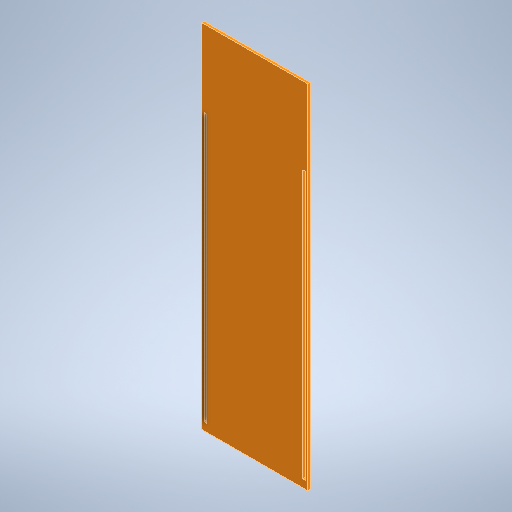
# Autodesk Inventor part: lifting cover 2
Saved by Autodesk Inventor 2025.4 (Build 294407000, 407)
## iProperties
Created: 2026-04-06
Part Number: lifting cover 2
Material: Generic
Document SubType Name: Modeling
Designer: abdo2
Density: 1 g/cm^3
Appearance: Orange
Author: abdo2
Autodesk Inventor part; units mm, degrees
ref_plane "YZ Plane" through (0, 0, 0) normal (1, 0, 0) x (0, 1, 0)
ref_plane "XZ Plane" through (0, 0, 0) normal (0, 1, 0) x (-1, 0, 0)
ref_plane "XY Plane" through (0, 0, 0) normal (0, 0, 1) x (1, 0, 0)
sketch "Sketch1" plane through (0, 0, 0) normal (0, 0, 1) x (1, 0, 0)
  line L0 (0, 0) -> (0, 439)
  line L1 (0, 439) -> (132, 439)
  line L2 (132, 439) -> (132, 0)
  line L3 (132, 0) -> (0, 0)
  line L4 (129, 343) -> (126, 343)
  line L5 (126, 343) -> (126, 10)
  line L6 (126, 10) -> (129, 10)
  line L7 (129, 10) -> (129, 343)
  line L8 (3, 343) -> (6, 343)
  line L9 (6, 343) -> (6, 10)
  line L10 (6, 10) -> (3, 10)
  line L11 (3, 10) -> (3, 343)
  dimension "d0" = 439
  dimension "d1" = 132
  dimension "d2" = 3
  dimension "d3" = 3
  dimension "d4" = 3
  dimension "d5" = 3
  dimension "d7" = 10
  dimension "d10" = 343
  constraints: 24 end point, 6 perpendicular, 3 point on line, 2 parallel, 1 vertical
  measures "d0" distance of L0.start L0.end
  measures "d1" distance of L0.end L1.end
  measures "d2" distance between parallel lines of L0 L11
  measures "d3" distance between parallel lines of L11 L9
  measures "d4" distance between parallel lines of L2 L7
  measures "d5" distance between parallel lines of L7 L5
  measures "d7" distance between parallel lines of L3 L6
  measures "d10" distance between parallel lines of L3 L8
extrude "Extrusion1" add sketch "Sketch1" along normal blind 3
body "Solid1"
